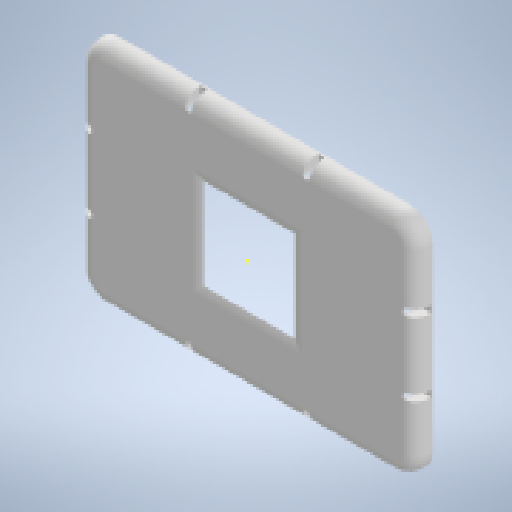
# Autodesk Inventor part: up
Saved by Autodesk Inventor 2025 (Build 290162000, 162)
## iProperties
Created: 2025-10-21
Part Number: up
Material: Generic
Document SubType Name: Modeling
Designer: hp
Density: 1 g/cm^3
Appearance: Default
Author: hp
Autodesk Inventor part; units mm, degrees
ref_plane "YZ Plane" through (0, 0, 0) normal (1, 0, 0) x (0, 1, 0)
ref_plane "XZ Plane" through (0, 0, 0) normal (0, 1, 0) x (-1, 0, 0)
ref_plane "XY Plane" through (0, 0, 0) normal (0, 0, 1) x (1, 0, 0)
sketch "Sketch1" plane through (0, 0, 0) normal (0, 0, 1) x (1, 0, 0)
  line L0 (-325, 254) -> (325, 254)
  line L1 (379, 200) -> (379, -200)
  line L2 (325, -254) -> (-325, -254)
  line L3 (-379, -200) -> (-379, 200)
  line L4 (-379, 254) -> (379, -254) construction
  line L5 (379, 254) -> (-379, -254) construction
  arc A0 (-325, 254) -> (-379, 200) centre (-325, 200) ccw
  arc A1 (379, 200) -> (325, 254) centre (325, 200) ccw
  arc A2 (325, -254) -> (379, -200) centre (325, -200) ccw
  arc A3 (-379, -200) -> (-325, -254) centre (-325, -200) ccw
  point P0 (0, 0)
  dimension "d0" = 758
  dimension "d1" = 508
  dimension "d2" = 54
  constraints: 12 end point, 8 point on circle, 8 point on line, 8 tangent, 4 centre point, 3 equal radius, 2 midpoint, 2 parallel, 1 horizontal, 1 perpendicular
  measures "d0" distance of L4.end L5.end
  measures "d1" distance of L5.start L4.end
  measures "d2" radius of A0
extrude "Extrusion1" add sketch "Sketch1" along normal blind 40
fillet "Fillet1" radius 30 8 edges at (-363.1838, 238.1838, 40) (-379, 0, 40) (-363.1838, -238.1838, 40) (0, -254, 40) (363.1838, -238.1838, 40) (379, 0, 40) (363.1838, 238.1838, 40) (0, 254, 40)
sketch "Sketch2" plane through (0, 0, 0) normal (0, 0, -1) x (-1, 0, 0)
  line L0 (294, 229) -> (-294, 229)
  line L1 (-354, 169) -> (-354, -169)
  line L2 (-294, -229) -> (294, -229)
  line L3 (354, -169) -> (354, 169)
  line L4 (354, 229) -> (-354, -229) construction
  line L5 (-354, 229) -> (354, -229) construction
  arc A0 (354, 169) -> (294, 229) centre (294, 169) ccw
  arc A1 (294, -229) -> (354, -169) centre (294, -169) ccw
  arc A2 (-354, -169) -> (-294, -229) centre (-294, -169) ccw
  arc A3 (-294, 229) -> (-354, 169) centre (-294, 169) ccw
  point P0 (0, 0)
  dimension "d6" = 708
  dimension "d7" = 458
  dimension "d8" = 60
  constraints: 12 end point, 8 point on circle, 8 point on line, 8 tangent, 4 centre point, 3 equal radius, 2 midpoint, 2 parallel, 1 horizontal, 1 perpendicular
  measures "d6" distance of L5.end L4.end
  measures "d7" distance of L5.end L4.start
  measures "d8" radius of A0
extrude "Extrusion2" cut sketch "Sketch2" against normal blind 35
sketch "Sketch3" plane through (0, 0, 40) normal (0, 0, 1) x (1, 0, 0)
  line L0 (-377.7666, 254) -> (272.2334, 254)
  line L1 (-140, 254) -> (-125, 254)
  line L2 (-125, -254) -> (-140, -254)
  line L3 (125, 254) -> (140, 254)
  line L4 (140, -254) -> (125, -254)
  line L5 (-379, -196) -> (-379, 204)
  line L6 (379, 86) -> (379, 71)
  line L7 (-379, 71) -> (-379, 86)
  line L8 (379, 224.0745) -> (379, -175.9255)
  line L9 (379, -79) -> (379, -94)
  line L10 (264.2334, -254) -> (-385.7666, -254)
  line L11 (125, 232.5) -> (125, 254)
  line L12 (140, 254) -> (140, 232.5)
  line L13 (-125, 254) -> (-125, 232.5)
  line L14 (-140, 232.5) -> (-140, 254)
  line L15 (-379, 86) -> (-357.5, 86)
  line L16 (-357.5, 71) -> (-379, 71)
  line L17 (-379, -79) -> (-357.5, -79)
  line L18 (-357.5, -94) -> (-435.7666, -94)
  line L19 (-140, -254) -> (-140, -232.5)
  line L20 (-125, -232.5) -> (-125, -254)
  line L21 (140, -232.5) -> (140, -254)
  line L22 (125, -254) -> (125, -232.5)
  line L23 (357.5, -79) -> (379, -79)
  line L24 (379, -94) -> (357.5, -94)
  line L25 (357.5, 86) -> (379, 86)
  line L26 (379, 71) -> (357.5, 71)
  arc A0 (-140, 232.5) -> (-125, 232.5) centre (-132.5, 232.5) ccw
  arc A1 (125, 232.5) -> (140, 232.5) centre (132.5, 232.5) ccw
  arc A2 (-357.5, 71) -> (-357.5, 86) centre (-357.5, 78.5) ccw
  arc A3 (-357.5, -94) -> (-357.5, -79) centre (-357.5, -86.5) ccw
  arc A4 (-125, -232.5) -> (-140, -232.5) centre (-132.5, -232.5) ccw
  arc A5 (140, -232.5) -> (125, -232.5) centre (132.5, -232.5) ccw
  arc A6 (357.5, -79) -> (357.5, -94) centre (357.5, -86.5) ccw
  arc A7 (357.5, 86) -> (357.5, 71) centre (357.5, 78.5) ccw
  circle A8 centre (132.5, 232.5) radius 2.5
  circle A9 centre (-132.5, 232.5) radius 2.5
  circle A10 centre (-357.5, 78.5) radius 2.5
  circle A11 centre (-357.5, -86.5) radius 2.5
  circle A12 centre (-132.5, -232.5) radius 2.5
  circle A13 centre (132.5, -232.5) radius 2.5
  circle A14 centre (357.5, -86.5) radius 2.5
  circle A15 centre (357.5, 78.5) radius 2.5
  line L27 (325, 254) -> (-325, 254) projected
  line L28 (-325, -254) -> (325, -254) projected
  line L29 (379, -200) -> (379, 200) projected
  line L30 (-379, 200) -> (-379, -200) projected
  line L31 (-102.5, -102.5) -> (102.5, -102.5)
  line L32 (102.5, -102.5) -> (102.5, 102.5)
  line L33 (102.5, 102.5) -> (-102.5, 102.5)
  line L34 (-102.5, 102.5) -> (-102.5, -102.5)
  line L35 (-102.5, -102.5) -> (102.5, 102.5) construction
  line L36 (102.5, -102.5) -> (-102.5, 102.5) construction
  point P0 (0, 0)
  point P1 (-132.5, -254)
  point P2 (132.5, -254)
  point P3 (-423.2666, 71)
  point P4 (301.7334, -79)
  point P5 (301.7334, 71)
  point P6 (301.7334, -94)
  point P7 (125, -163.4255)
  point P8 (-140, -163.4255)
  point P9 (-379, 78.5)
  point P10 (-132.5, -225)
  point P11 (379, -86.5)
  point P12 (-379, -94)
  dimension "d11" = 758
  dimension "d12" = 15
  dimension "d13" = 0
  dimension "d14" = 250
  dimension "d15" = 239
  dimension "d16" = 15
  dimension "d17" = 15
  dimension "d18" = 150
  dimension "d19" = 160
  dimension "d20" = 15
  dimension "d21" = 150
  dimension "d22" = 160
  dimension "d23" = 15
  dimension "d24" = 15
  dimension "d25" = 254
  dimension "d26" = 250
  dimension "d27" = 15
  dimension "d28" = 5
  dimension "d29" = 5
  dimension "d30" = 5
  dimension "d31" = 5
  dimension "d32" = 5
  dimension "d33" = 5
  dimension "d34" = 5
  dimension "d35" = 5
  dimension "d36" = 21.5
  dimension "d37" = 21.5
  dimension "d38" = 21.5
  dimension "d39" = 15
  dimension "d40" = 21.5
  dimension "d41" = 21.5
  dimension "d42" = 29
  dimension "d43" = 21.5
  dimension "d44" = 21.5
  dimension "d83" = 205
  dimension "d84" = 205
  dimension "d87" = 150
  constraints: 66 end point, 21 parallel, 17 point on circle, 16 centre point, 16 tangent, 12 point on line, 9 perpendicular, 8 coincident, 7 horizontal, 6 midpoint, 5 collinear
  measures "d11" distance of L15.start L6.start
  measures "d12" distance of L6.start L6.end
  measures "d13" distance from line of L10 point (-132.5, -254)
  measures "d14" distance from line of L3.start L13
  measures "d15" distance between parallel lines of L8 L12
  measures "d16" distance from line of L3.end L11
  measures "d17" distance between parallel lines of L16 L15
  measures "d18" distance from line of L17 point (-423.267, 71)
  measures "d19" distance between parallel lines of L10 L18
  measures "d20" distance between parallel lines of L18 L17
  measures "d21" distance of point (301.733, -79) point (301.733, 71)
  measures "d22" distance from line of L10 point (301.733, -94)
  measures "d23" distance between parallel lines of L24 L23
  measures "d24" distance from line of point (125, -163.426) L21
  measures "d25" distance from line of L8 point (125, -163.426)
  measures "d26" distance between parallel lines of L22 L20
  measures "d27" distance from line of L20 point (-140, -163.426)
  measures "d28" diameter of A8
  measures "d29" diameter of A9
  measures "d30" diameter of A10
  measures "d31" diameter of A11
  measures "d32" diameter of A12
  measures "d33" diameter of A13
  measures "d34" diameter of A14
  measures "d35" diameter of A15
  measures "d36" distance from line of L4 A5.centre
  measures "d37" distance from line of A1.centre L3
  measures "d38" distance from line of A0.centre L0
  measures "d39" distance between parallel lines of L13 L14
  measures "d40" distance of point (-379, 78.5) A2.centre
  measures "d41" distance from line of L5 A3.centre
  measures "d42" distance from line of L10 point (-132.5, -225)
  measures "d43" distance of point (379, -86.5) A6.centre
  measures "d44" distance from line of A7.centre L6
  measures "d83" distance of L33.end L32.end
  measures "d84" distance of L32.end L31.end
  measures "d87" distance between parallel lines of L23 L26
sketch "Sketch4" plane through (0, 0, 0) normal (0, 0, -1) x (-1, 0, 0)
  line L0 (-329.5439, 254) -> (320.4561, 254)
  line L1 (-140, 254) -> (-125, 254)
  line L2 (-125, -254) -> (-140, -254)
  line L3 (125, 254) -> (140, 254)
  line L4 (140, -254) -> (125, -254)
  line L5 (-379, -204) -> (-379, 196)
  line L6 (379, 86) -> (379, 71)
  line L7 (-379, 71) -> (-379, 86)
  line L8 (379, 206.0747) -> (379, -193.9253)
  line L9 (379, -79) -> (379, -94)
  line L10 (328.4561, -254) -> (-321.5439, -254)
  line L11 (125, 232.5) -> (125, 254)
  line L12 (140, 254) -> (140, 232.5)
  line L13 (-125, 254) -> (-125, 232.5)
  line L14 (-140, 232.5) -> (-140, 254)
  line L15 (-379, 86) -> (-357.5, 86)
  line L16 (-357.5, 71) -> (-379, 71)
  line L17 (-379, -79) -> (-357.5, -79)
  line L18 (-357.5, -94) -> (-371.5439, -94)
  line L19 (-140, -254) -> (-140, -232.5)
  line L20 (-125, -232.5) -> (-125, -254)
  line L21 (140, -232.5) -> (140, -254)
  line L22 (125, -254) -> (125, -232.5)
  line L23 (357.5, -79) -> (379, -79)
  line L24 (379, -94) -> (357.5, -94)
  line L25 (357.5, 86) -> (379, 86)
  line L26 (379, 71) -> (357.5, 71)
  arc A0 (-140, 232.5) -> (-125, 232.5) centre (-132.5, 232.5) ccw
  arc A1 (125, 232.5) -> (140, 232.5) centre (132.5, 232.5) ccw
  arc A2 (-357.5, 71) -> (-357.5, 86) centre (-357.5, 78.5) ccw
  arc A3 (-357.5, -94) -> (-357.5, -79) centre (-357.5, -86.5) ccw
  arc A4 (-125, -232.5) -> (-140, -232.5) centre (-132.5, -232.5) ccw
  arc A5 (140, -232.5) -> (125, -232.5) centre (132.5, -232.5) ccw
  arc A6 (357.5, -79) -> (357.5, -94) centre (357.5, -86.5) ccw
  arc A7 (357.5, 86) -> (357.5, 71) centre (357.5, 78.5) ccw
  circle A8 centre (132.5, 232.5) radius 2.5
  circle A9 centre (-132.5, 232.5) radius 2.5
  circle A10 centre (-357.5, 78.5) radius 2.5
  circle A11 centre (-357.5, -86.5) radius 2.5
  circle A12 centre (-132.5, -232.5) radius 2.5
  circle A13 centre (132.5, -232.5) radius 2.5
  circle A14 centre (357.5, -86.5) radius 2.5
  circle A15 centre (357.5, 78.5) radius 2.5
  line L27 (325, -254) -> (-325, -254) projected
  line L28 (379, 200) -> (379, -200) projected
  line L29 (-379, -200) -> (-379, 200) projected
  line L30 (-325, 254) -> (325, 254) projected
  point P0 (0, 0)
  point P1 (-132.5, -254)
  point P2 (132.5, -254)
  point P3 (-359.0439, 71)
  point P4 (365.9561, -79)
  point P5 (365.9561, 71)
  point P6 (365.9561, -94)
  point P7 (125, -181.4253)
  point P8 (-140, -181.4253)
  point P9 (-379, 78.5)
  point P10 (-132.5, -225)
  point P11 (379, -86.5)
  dimension "d45" = 758
  dimension "d46" = 15
  dimension "d47" = 0
  dimension "d48" = 250
  dimension "d49" = 239
  dimension "d50" = 15
  dimension "d51" = 15
  dimension "d52" = 150
  dimension "d53" = 160
  dimension "d54" = 15
  dimension "d55" = 150
  dimension "d56" = 160
  dimension "d57" = 15
  dimension "d58" = 15
  dimension "d59" = 254
  dimension "d60" = 250
  dimension "d61" = 15
  dimension "d62" = 5
  dimension "d63" = 5
  dimension "d64" = 5
  dimension "d65" = 5
  dimension "d66" = 5
  dimension "d67" = 5
  dimension "d68" = 5
  dimension "d69" = 5
  dimension "d70" = 21.5
  dimension "d71" = 21.5
  dimension "d72" = 21.5
  dimension "d73" = 15
  dimension "d74" = 21.5
  dimension "d75" = 21.5
  dimension "d76" = 29
  dimension "d77" = 21.5
  dimension "d78" = 21.5
  constraints: 54 end point, 19 parallel, 17 point on circle, 16 centre point, 16 tangent, 12 point on line, 8 coincident, 8 perpendicular, 6 horizontal, 5 collinear, 4 midpoint
  measures "d45" distance of L15.start L25.end
  measures "d46" distance of L25.end L6.end
  measures "d47" distance from line of L10 point (-132.5, -254)
  measures "d48" distance from line of L3.start L13
  measures "d49" distance between parallel lines of L8 L12
  measures "d50" distance from line of L12.start L11
  measures "d51" distance between parallel lines of L16 L15
  measures "d52" distance from line of L17 point (-359.044, 71)
  measures "d53" distance between parallel lines of L10 L18
  measures "d54" distance between parallel lines of L18 L17
  measures "d55" distance of point (365.956, -79) point (365.956, 71)
  measures "d56" distance from line of L10 point (365.956, -94)
  measures "d57" distance between parallel lines of L24 L23
  measures "d58" distance from line of point (125, -181.425) L21
  measures "d59" distance from line of L8 point (125, -181.425)
  measures "d60" distance between parallel lines of L22 L20
  measures "d61" distance from line of L20 point (-140, -181.425)
  measures "d62" diameter of A8
  measures "d63" diameter of A9
  measures "d64" diameter of A10
  measures "d65" diameter of A11
  measures "d66" diameter of A12
  measures "d67" diameter of A13
  measures "d68" diameter of A14
  measures "d69" diameter of A15
  measures "d70" distance from line of L4 A5.centre
  measures "d71" distance from line of A1.centre L3
  measures "d72" distance from line of A0.centre L0
  measures "d73" distance between parallel lines of L13 L14
  measures "d74" distance of point (-379, 78.5) A2.centre
  measures "d75" distance from line of L5 A3.centre
  measures "d76" distance from line of L10 point (-132.5, -225)
  measures "d77" distance of point (379, -86.5) A6.centre
  measures "d78" distance from line of A7.centre L6
extrude "Extrusion3" cut sketch "Sketch3" against normal blind 35 contours L0 L13 A0 L14 | L0 L12 A1 L11 | L2 L19 A4 L20 | L4 L22 A5 L21 | L5 L15 A2 L16 | L5 L17 A3 L18 | L6 L26 A7 L25 | L8 L24 A6 L23 | A13
extrude "Extrusion4" cut sketch "Sketch3" against normal through all contours A8 | A9 | A10 | A11 | A12 | A13 | A14 | A15
extrude "Extrusion5" cut sketch "Sketch3" against normal blind 10 contours L34 L33 L32 L31
fillet "Fillet2" radius 40 4 edges at (102.5, 0, 40) (0, -102.5, 40) (-102.5, 0, 40) (0, 102.5, 40)
sketch "Sketch5" plane through (0, 0, 40) normal (0, 0, 1) x (1, 0, 0)
  point P0 (0, 0)
body "Solid1"
